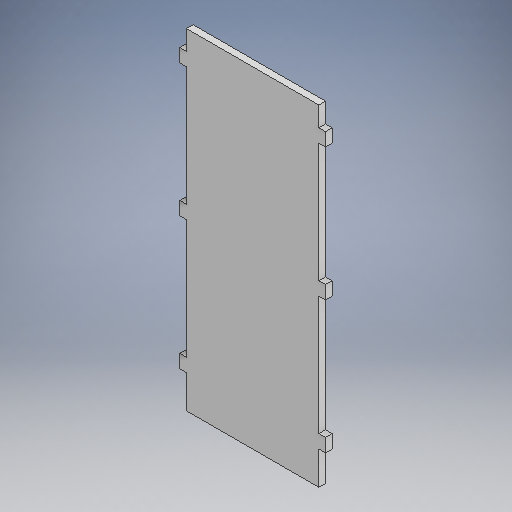
# Autodesk Inventor part: Lifting Sections all back
Saved by Autodesk Inventor 2025.3 (Build 293356000, 356)
## iProperties
Created: 2026-04-06
Part Number: Lifting Sections all back
Material: Generic
Document SubType Name: Modeling
Designer: user
Density: 1 g/cm^3
Appearance: Default
Author: user
Autodesk Inventor part; units mm, degrees
ref_plane "YZ Plane" through (0, 0, 0) normal (1, 0, 0) x (0, 1, 0)
ref_plane "XZ Plane" through (0, 0, 0) normal (0, 1, 0) x (-1, 0, 0)
ref_plane "XY Plane" through (0, 0, 0) normal (0, 0, 1) x (1, 0, 0)
sketch "Sketch1" plane through (0, 0, 0) normal (0, 0, 1) x (1, 0, 0)
  line L0 (-61.8393, -52.0586) -> (-61.8393, 197.9414)
  line L1 (-11.8393, -52.0586) -> (-11.8393, 197.9414) construction
  line L2 (38.1607, -52.0586) -> (38.1607, 145.9423)
  line L3 (38.1607, -52.0586) -> (-61.8393, -52.0586)
  line L4 (43.1607, 183.0414) -> (38.1607, 183.0414)
  line L5 (43.1607, 172.9414) -> (43.1607, 183.0414)
  line L6 (38.1607, 172.9414) -> (43.1607, 172.9414)
  line L7 (43.1607, -16.9586) -> (38.1607, -16.9586)
  line L8 (43.1607, -27.0586) -> (43.1607, -16.9586)
  line L9 (38.1607, -27.0586) -> (43.1607, -27.0586)
  line L10 (-61.8393, 83.0414) -> (-61.8393, 72.9414)
  line L11 (-61.8393, 72.9414) -> (38.1607, 72.9414) construction
  line L12 (38.1607, 72.9414) -> (43.1607, 72.9414)
  line L13 (38.1607, 72.9414) -> (43.1607, 72.9414)
  line L14 (43.1607, 72.9414) -> (43.1607, 83.0414)
  line L15 (43.1607, 72.9414) -> (43.1607, 83.0414)
  line L16 (43.1607, 83.0414) -> (38.1607, 83.0414)
  line L17 (43.1607, 83.0414) -> (38.1607, 83.0414)
  line L18 (38.1607, 145.9423) -> (38.1607, 197.9414)
  line L19 (38.1607, 197.9414) -> (38.1607, 147.9414)
  line L20 (38.1607, 147.9414) -> (-61.8393, 147.9414) construction
  line L21 (-66.8393, -27.0586) -> (-66.8393, -16.9586)
  line L22 (-66.8393, -16.9586) -> (-61.8393, -16.9586)
  line L23 (-61.8393, -27.0586) -> (-66.8393, -27.0586)
  line L24 (-66.8393, 83.0414) -> (-61.8393, 83.0414)
  line L25 (-66.8393, 72.9414) -> (-66.8393, 83.0414)
  line L26 (-61.8393, 72.9414) -> (-66.8393, 72.9414)
  line L27 (-66.8393, 172.9414) -> (-66.8393, 183.0414)
  line L28 (-66.8393, 183.0414) -> (-61.8393, 183.0414)
  line L29 (-61.8393, 172.9414) -> (-66.8393, 172.9414)
  line L30 (-61.8393, 197.9414) -> (38.1607, 197.9414)
  line L31 (38.1607, 197.9414) -> (28.1607, 197.9414)
  line L32 (38.1607, 149.2033) -> (38.1607, 197.9414)
  line L33 (-61.8393, 197.9414) -> (-51.8393, 197.9414)
  line L34 (-61.8393, 149.2728) -> (-61.8393, 197.9414)
  line L35 (-61.8393, 147.9414) -> (38.1607, 147.9414) construction
  line L36 (28.1607, 145.2728) -> (28.1607, 139.2728)
  line L37 (17.1607, 145.2728) -> (17.1607, 139.2728)
  line L38 (-40.8393, 145.2728) -> (-40.8393, 139.2728)
  line L39 (-51.8393, 145.2728) -> (-51.8393, 139.2728)
  line L40 (17.1607, 145.2728) -> (-40.8393, 145.2728) construction
  line L41 (17.1607, 139.2728) -> (-40.8393, 139.2728) construction
  line L42 (28.1607, 139.2728) -> (17.1607, 139.2728)
  line L43 (28.1607, 145.2728) -> (17.1607, 145.2728)
  line L44 (-40.8393, 145.2728) -> (-51.8393, 145.2728)
  line L45 (-40.8393, 139.2728) -> (-51.8393, 139.2728)
  line L46 (-51.8393, 139.2728) -> (-61.8393, 139.2728) construction
  line L47 (-51.8393, 145.2728) -> (-61.8393, 145.2728) construction
  dimension "d8" = 10
  dimension "d9" = 11
  constraints: 96 end point, 12 perpendicular, 6 symmetric about line, 5 point on line, 2 horizontal, 1 vertical
  measures "d8" distance between parallel lines of L2 L36
  measures "d9" distance between parallel lines of L37 L36
extrude "Extrusion1" add sketch "Sketch1" along normal blind 5 contours L0 L30 L18 L2 L3 | L23 L21 L22 L0 | L2 L7 L8 L9 | L26 L25 L24 L0 | L2 L16 L14 L12 | L29 L27 L28 L0 | L18 L4 L5 L6 | L36 L42 L37 L43 | L38 L45 L39 L44
body "Solid1"
